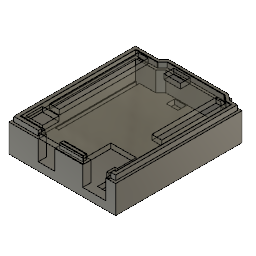
Boîte Arduino V2 F3D (Autodesk Fusion 360 design; units mm, degrees)
Autodesk Fusion 360 part; units mm, degrees
sketch "Esquisse1" plane through (0, 0, 0) normal (0, 0, 1) x (1, 0, 0) in component "Boîte"
  line L0 (-80.3671, -46.9664) -> (-25.3671, -46.9664)
  line L1 (-25.3671, -46.9664) -> (-25.3671, 20.0336)
  line L2 (-80.3671, -46.9664) -> (-80.3671, 20.0336)
  line L3 (-25.3671, 20.0336) -> (-27.7671, 20.0336)
  line L4 (-31.5449, 23.0558) -> (-64.9449, 23.0558)
  line L5 (-67.9671, 20.0336) -> (-80.3671, 20.0336)
  line L6 (-64.9449, 23.0558) -> (-67.9671, 20.0336)
  line L7 (-31.5449, 23.0558) -> (-27.7671, 20.0336)
  line L8 (-85.3671, 25.0336) -> (-85.3671, -51.9664)
  line L9 (-85.3671, -51.9664) -> (-20.3671, -51.9664)
  line L10 (-20.3671, -51.9664) -> (-20.3671, 25.0336)
  line L11 (-20.3671, 25.0336) -> (-26.0132, 25.0336)
  line L12 (-26.0132, 25.0336) -> (-29.791, 28.0558)
  line L13 (-29.791, 28.0558) -> (-67.016, 28.0558)
  line L14 (-67.016, 28.0558) -> (-70.0382, 25.0336)
  line L15 (-70.0382, 25.0336) -> (-85.3671, 25.0336)
  dimension "larg" = 55
  dimension "long" = 67
  dimension "d10" = 67
  dimension "petitcoin" = 2.4
  dimension "d15" = 33.4
  dimension "d18" = 12.4
  dimension "ep" = 5
  dimension "d21" = 5
  dimension "d22" = 5
  dimension "d24" = 5
  dimension "d25" = 5
  dimension "d26" = 5
  dimension "d27" = 5
  dimension "d28" = 5
  constraint horizontal L0
  constraint perpendicular L0 L1
  constraint perpendicular L0 L2
  constraint perpendicular L1 L3
  constraint perpendicular L2 L5
  constraint vertical L8
  constraint perpendicular L8 L9
  constraint perpendicular L9 L10
  constraint perpendicular L10 L11
  constraint perpendicular L10 L13
  constraint perpendicular L8 L15
  constraint parallel L6 L14
  constraint parallel L4 L13
  constraint parallel L7 L12
  measures "larg" distance of L0.start L0.end
  measures "long" distance of L0.end L1.end
  measures "d10" distance of L0.start L2.end
  measures "petitcoin" distance of L1.end L3.end
  measures "d15" distance of L4.start L4.end
  measures "d18" distance of L5.start L2.end
  measures "ep" distance of L2 L8
  measures "d21" distance of L1 L10
  measures "d22" distance of L0 L9
  measures "d24" distance of L6 L14
  measures "d25" distance of L7 L12
  measures "d26" distance of L3 L11
  measures "d27" distance of L4 L13
  measures "d28" distance of L5 L15
sketch "Esquisse2" plane through (0, 0, 0) normal (0, 0, 1) x (1, 0, 0) in component "Boîte"
  line L0 (-26.3671, -46.9664) -> (-40.3671, -46.9664)
  line L1 (-57.3671, -46.9664) -> (-67.3671, -46.9664)
  line L2 (-67.3671, -46.9664) -> (-67.3671, -51.9664)
  line L3 (-57.3671, -46.9664) -> (-57.3671, -51.9664)
  line L4 (-67.3671, -51.9664) -> (-57.3671, -51.9664)
  line L5 (-40.3671, -46.9664) -> (-40.3671, -51.9664)
  line L6 (-26.3671, -46.9664) -> (-26.3671, -51.9664)
  line L7 (-40.3671, -51.9664) -> (-26.3671, -51.9664)
  line L8 (-25.3671, -46.9664) -> (-25.3671, -35.9664)
  line L9 (-25.3671, -35.9664) -> (-36.3671, -35.9664)
  line L10 (-36.3671, -35.9664) -> (-36.3671, -46.9664)
  line L11 (-36.3671, -46.9664) -> (-25.3671, -46.9664)
  line L12 (-25.3671, 20.0336) -> (-25.8671, 20.0336)
  line L13 (-25.8671, 20.0336) -> (-27.8671, 20.0336)
  line L14 (-25.8671, 20.0336) -> (-25.8671, -19.9664)
  line L15 (-27.8671, 20.0336) -> (-27.8671, -19.9664)
  line L16 (-27.8671, -19.9664) -> (-25.8671, -19.9664)
  line L17 (-80.3671, 20.0336) -> (-79.8671, 20.0336)
  line L18 (-79.8671, 20.0336) -> (-77.8671, 20.0336)
  line L19 (-79.8671, 20.0336) -> (-79.8671, -28.9664)
  line L20 (-77.8671, 20.0336) -> (-77.8671, -28.9664)
  line L21 (-79.8671, -28.9664) -> (-77.8671, -28.9664)
  line L22 (-59, 22.5) -> (-52, 22.5)
  line L23 (-59, 22.5) -> (-59, 17.5)
  line L24 (-59, 17.5) -> (-52, 17.5)
  line L25 (-52, 17.5) -> (-52, 22.5)
  point P0 (-25.3671, -46.9664)
  point P1 (-25.3671, 20.0336)
  point P2 (-80.3671, 20.0336)
  dimension "d29" = 1
  dimension "d30" = 14
  dimension "d31" = 17
  dimension "d32" = 10
  dimension "d33" = 5
  dimension "d34" = 5
  dimension "d35" = 5
  dimension "d36" = 5
  dimension "d37" = 11
  dimension "d38" = 11
  dimension "d39" = 11
  dimension "d40" = 0.5
  dimension "d41" = 2
  dimension "d42" = 40
  dimension "d43" = 40
  dimension "d44" = 0.5
  dimension "d45" = 2
  dimension "d46" = 49
  dimension "d47" = 49
  dimension "d50" = 7
  dimension "d51" = 5
  constraint horizontal L0
  constraint perpendicular L1 L2
  constraint perpendicular L1 L3
  constraint perpendicular L0 L5
  constraint perpendicular L0 L6
  constraint coincident P0 L8.start
  constraint perpendicular L7 L8
  constraint perpendicular L8 L9
  constraint perpendicular L9 L10
  constraint coincident P1 L12.start
  constraint horizontal L12
  constraint parallel L12 L13
  constraint perpendicular L12 L14
  constraint perpendicular L13 L15
  constraint coincident P2 L17.start
  constraint horizontal L17
  constraint horizontal L18
  constraint perpendicular L17 L19
  constraint perpendicular L18 L20
  constraint perpendicular L22 L23
  constraint perpendicular L23 L24
  measures "d29" distance of P0 L0.start
  measures "d30" distance of L0.start L0.end
  measures "d31" distance of L0.end L1.start
  measures "d32" distance of L1.start L1.end
  measures "d33" distance of L1.end L2.end
  measures "d34" distance of L1.start L3.end
  measures "d35" distance of L0.end L5.end
  measures "d36" distance of L0.start L6.end
  measures "d37" distance of P0 L8.end
  measures "d38" distance of L8.end L9.end
  measures "d39" distance of L9.end L10.end
  measures "d40" distance of P1 L12.end
  measures "d41" distance of L12.end L13.end
  measures "d42" distance of L12.end L14.end
  measures "d43" distance of L13.end L15.end
  measures "d44" distance of P2 L17.end
  measures "d45" distance of L17.end L18.end
  measures "d46" distance of L17.end L19.end
  measures "d47" distance of L18.end L20.end
  measures "d50" distance of L22.start L22.end
  measures "d51" distance of L22.start L23.end
extrude "Extrusion3" add sketch "Esquisse1" against normal blind 5 contours L0 L1 L2 L3 L4 L5 L6 L7 makes body 1 in component "Boîte"
extrude "Extrusion5" cut sketch "Esquisse2" against normal blind 3 contours L0 L8 L9 L10 L11 | L13 L14 L15 L16 | L18 L19 L20 L21 | L22 L23 L24 L25 bodies 1 in component "Boîte"
extrude "Extrusion6" add sketch "Esquisse1" against normal blind 5 bodies 1 in component "Boîte"
extrude "Extrusion7" add sketch "Esquisse1" along normal blind 12 bodies 1 in component "Boîte"
extrude "Extrusion8" cut sketch "Esquisse2" along normal blind 15 contours L0 L5 L6 L7 L11 | L1 L2 L3 L4 bodies 1 in component "Boîte"
sketch "Esquisse1 (2)" plane through (0, 0, 12) normal (0, 0, 1) x (-1, 0, 0)
  line L0 (67.3671, 51.9664) -> (67.3671, 46.9664)
  line L1 (67.3671, 46.9664) -> (80.3671, 46.9664)
  line L2 (80.3671, 46.9664) -> (80.3671, -20.0336)
  line L3 (80.3671, -20.0336) -> (67.9671, -20.0336)
  line L4 (67.9671, -20.0336) -> (64.9449, -23.0558)
  line L5 (64.9449, -23.0558) -> (31.5449, -23.0558)
  line L6 (31.5449, -23.0558) -> (27.7671, -20.0336)
  line L7 (27.7671, -20.0336) -> (25.3671, -20.0336)
  line L8 (25.3671, -20.0336) -> (25.3671, 46.9664)
  line L9 (25.3671, 46.9664) -> (26.3671, 46.9664)
  line L10 (26.3671, 46.9664) -> (26.3671, 51.9664)
  line L11 (26.3671, 51.9664) -> (20.3671, 51.9664)
  line L12 (20.3671, 51.9664) -> (20.3671, -25.0336)
  line L13 (20.3671, -25.0336) -> (26.0132, -25.0336)
  line L14 (26.0132, -25.0336) -> (29.791, -28.0558)
  line L15 (29.791, -28.0558) -> (67.016, -28.0558)
  line L16 (67.016, -28.0558) -> (70.0382, -25.0336)
  line L17 (70.0382, -25.0336) -> (85.3671, -25.0336)
  line L18 (85.3671, -25.0336) -> (85.3671, 51.9664)
  line L19 (85.3671, 51.9664) -> (67.3671, 51.9664)
  line L20 (83.8671, -20) -> (83.8671, 47)
  line L21 (81.8671, 47) -> (81.8671, -20)
  line L22 (83.8671, 47) -> (83.8671, 50.4664)
  line L23 (83.8671, 50.4664) -> (68.8671, 50.4664)
  line L24 (68.8671, 50.4664) -> (68.8671, 48.4664)
  line L25 (68.8671, 48.4664) -> (81.8671, 48.4664)
  line L26 (81.8671, 48.4664) -> (81.8671, 47)
  line L27 (55.8671, 50.4664) -> (41.8671, 50.4664)
  line L28 (41.8671, 50.4664) -> (41.8671, 48.4664)
  line L29 (41.8671, 48.4664) -> (55.8671, 48.4664)
  line L30 (55.8671, 48.4664) -> (55.8671, 50.4664)
  line L31 (24.8671, 48.4664) -> (24.8671, 50.4664)
  line L32 (24.8671, 50.4664) -> (21.8671, 50.4664)
  line L33 (21.8671, 50.4664) -> (21.8671, -23.5336)
  line L34 (21.8671, -23.5336) -> (26.5394, -23.5336)
  line L35 (26.5394, -23.5336) -> (30.3172, -26.5558)
  line L36 (30.3172, -26.5558) -> (66.3946, -26.5558)
  line L37 (66.3946, -26.5558) -> (69.4169, -23.5336)
  line L38 (69.4169, -23.5336) -> (83.8671, -23.5336)
  line L39 (83.8671, -23.5336) -> (83.8671, -20)
  line L40 (81.8671, -20) -> (81.8671, -21.5336)
  line L41 (81.8671, -21.5336) -> (68.5884, -21.5336)
  line L42 (68.5884, -21.5336) -> (65.5662, -24.5558)
  line L43 (65.5662, -24.5558) -> (31.0187, -24.5558)
  line L44 (31.0187, -24.5558) -> (27.2409, -21.5336)
  line L45 (27.2409, -21.5336) -> (23.8671, -21.5336)
  line L46 (23.8671, -21.5336) -> (23.8671, 48.4664)
  line L47 (23.8671, 48.4664) -> (24.8671, 48.4664)
  line L48 (67.3671, 46.9664) -> (67.3671, 51.9664)
  line L49 (67.3671, 51.9664) -> (57.3671, 51.9664)
  line L50 (57.3671, 46.9664) -> (67.3671, 46.9664)
  line L51 (57.3671, 46.9664) -> (57.3671, 51.9664)
  line L52 (40.3671, 46.9664) -> (40.3671, 51.9664)
  line L53 (26.3671, 46.9664) -> (26.3671, 51.9664)
  line L54 (25.3671, 46.9664) -> (25.3671, 35.9664)
  line L55 (36.3671, 46.9664) -> (25.3671, 46.9664)
  line L56 (25.3671, -20.0336) -> (25.8671, -20.0336)
  dimension "d68" = 1.5
  dimension "distancebord" = 1.5
  dimension "d70" = 1.5
  dimension "d71" = 1.5
  dimension "d72" = 1.5
  dimension "d73" = 1.5
  dimension "d74" = 1.5
  dimension "d75" = 1.5
  dimension "d76" = 1.5
  dimension "d77" = 1.5
  dimension "d78" = 1.5
  dimension "d79" = 1.5
  dimension "d80" = 1.5
  dimension "d81" = 1.5
  dimension "d82" = 1.5
  dimension "d83" = 1.5
  dimension "d84" = 1.5
  dimension "d85" = 1.5
  dimension "d86" = 1.5
  dimension "d87" = 1.5
  dimension "d88" = 1.5
  dimension "d89" = 1.5
  dimension "d90" = 1.5
  dimension "d91" = 1.5
  constraint perpendicular L19 L20
  constraint perpendicular L3 L21
  constraint perpendicular L22 L23
  constraint perpendicular L23 L24
  constraint perpendicular L22 L25
  constraint perpendicular L27 L28
  constraint perpendicular L27 L30
  constraint perpendicular L27 L31
  constraint perpendicular L31 L32
  constraint perpendicular L33 L34
  constraint parallel L17 L36
  constraint parallel L3 L38
  constraint perpendicular L21 L41
  constraint perpendicular L20 L43
  constraint perpendicular L8 L45
  constraint perpendicular L45 L46
  constraint parallel L32 L47
  constraint parallel L12 L33
  constraint parallel L14 L35
  constraint parallel L6 L44
  constraint parallel L16 L37
  constraint parallel L4 L42
  measures "d68" distance of L18 L20
  measures "distancebord" distance of L2 L21
  measures "d70" distance of L1 L25
  measures "d71" distance of L19 L23
  measures "d72" distance of L24 L48
  measures "d73" distance of L27 L49
  measures "d74" distance of L29 L50
  measures "d75" distance of L30 L51
  measures "d76" distance of L28 L52
  measures "d77" distance of L31 L53
  measures "d78" distance of L11 L32
  measures "d79" distance of L12 L33
  measures "d80" distance of L46 L54
  measures "d81" distance of L47 L55
  measures "d82" distance of L13 L34
  measures "d83" distance of L45 L56
  measures "d84" distance of L14 L35
  measures "d85" distance of L6 L44
  measures "d86" distance of L15 L36
  measures "d87" distance of L5 L43
  measures "d88" distance of L16 L37
  measures "d89" distance of L4 L42
  measures "d90" distance of L17 L38
  measures "d91" distance of L3 L41
extrude "Extrusion9" add sketch "Esquisse1 (2)" along normal blind 3 contours L20 L21 L22 L23 L24 L25 L26 L31 L32 L33 L34 L35 L36 L37 L38 L39 L40 L41 L42 L43 L44 L45 L46 L47 | L27 L28 L29 L30 bodies 1 in component "Boîte"
sketch "Esquisse1 (3)" plane through (0, 0, 0) normal (0, 0, 1) x (1, 0, 0) in component "Couvercle"
  line L0 (35.6322, 76.6557) -> (35.6322, 78.6557)
  line L1 (35.6322, 76.6556) -> (35.6322, 78.6559)
  line L2 (4.6323, 75.1557) -> (6.1323, 75.1557)
  line L3 (48.3868, 6.6882) -> (61.6322, 6.6882)
  line L4 (6.1323, 75.1557) -> (6.1323, 80.1558)
  line L5 (3.6323, 76.6) -> (4.7432, 76.6)
  line L6 (7.0061, 6.6549) -> (10.7839, 3.6333)
  line L7 (35.6322, 76.6556) -> (21.6323, 76.6556)
  line L8 (4.7432, 76.6) -> (4.7432, 80.1428)
  line L9 (61.6322, 6.6882) -> (61.6322, 76.5747)
  line L10 (21.6323, 78.6557) -> (21.6323, 76.6557)
  line L11 (50.1322, 75.1557) -> (60.1322, 75.1557)
  line L12 (21.6323, 78.6559) -> (21.6323, 76.6556)
  line L13 (12.1323, 7.6894) -> (6.1323, 7.6894)
  line L14 (12.1323, 46.6558) -> (12.1323, 7.6894)
  line L15 (47.1323, 80.1558) -> (47.1323, 76.5747)
  line L16 (35.6322, 78.6559) -> (21.6323, 78.6559)
  line L17 (3.6323, 6.6549) -> (7.0061, 6.6549)
  line L18 (50.1322, 65.1557) -> (50.1322, 75.1557)
  line L19 (40.3313, 5.1336) -> (30.3313, 5.1336)
  line L20 (30.3313, 5.1336) -> (30.3313, 11.1336)
  line L21 (6.1323, 7.6894) -> (6.1323, 46.6558)
  line L22 (45.3312, 3.6333) -> (48.3868, 6.6882)
  line L23 (53.3822, 7.6894) -> (59.3822, 7.6894)
  line L24 (35.6322, 78.6557) -> (21.6323, 78.6557)
  line L25 (21.6323, 76.6556) -> (35.6322, 76.6556)
  line L26 (60.1322, 65.1557) -> (50.1322, 65.1557)
  line L27 (30.3313, 11.1336) -> (40.3313, 11.1336)
  line L28 (47.1323, 80.1558) -> (4.7432, 80.1558)
  line L29 (21.6323, 76.6557) -> (35.6322, 76.6557)
  line L30 (53.3822, 61.6557) -> (53.3822, 7.6894)
  line L31 (10.7838, 3.6333) -> (45.3312, 3.6333)
  line L32 (20.1324, 78.6559) -> (20.1324, 80.1558)
  line L33 (3.6323, 76.6) -> (3.6323, 6.6549)
  line L34 (40.3313, 11.1336) -> (40.3313, 5.1336)
  line L35 (47.1323, 76.5747) -> (61.6322, 76.5747)
  line L36 (4.6323, 63.6558) -> (4.6323, 75.1557)
  line L37 (35.6322, 76.6556) -> (35.6322, 78.6559)
  line L38 (60.1322, 75.1557) -> (60.1322, 65.1557)
  line L39 (59.3822, 61.6557) -> (53.3822, 61.6557)
  line L40 (20.1324, 78.6559) -> (20.1324, 63.6558)
  line L41 (6.1323, 46.6558) -> (12.1323, 46.6558)
  line L42 (59.3822, 7.6894) -> (59.3822, 61.6557)
  line L43 (20.1324, 63.6558) -> (4.6323, 63.6558)
  constraint coincident L2.start L36
  constraint perpendicular L2 L36
  constraint perpendicular L5 L8
  constraint perpendicular L15 L28
  constraint coincident L15 L35.start
  constraint perpendicular L15 L35
  constraint coincident L9 L35.end
  constraint perpendicular L9 L35
  constraint perpendicular L17 L33
  constraint perpendicular L3 L9
sketch "Esquisse2 (2)" plane through (0, 0, 0) normal (0, 0, 1) x (1, 0, 0) in component "Couvercle"
  line L0 (4.7432, 76.6) -> (4.7432, 80.1428)
  line L1 (4.7432, 80.1428) -> (20.1324, 80.1558)
  line L2 (20.1324, 80.1558) -> (20.1324, 63.6558)
  line L3 (20.1324, 63.6558) -> (4.6323, 63.6558)
  line L4 (20.1324, 80.1558) -> (21.6323, 80.1571)
  line L5 (21.6323, 80.1571) -> (47.1323, 80.1558)
  line L6 (47.1323, 80.1558) -> (47.1323, 76.5747)
  line L7 (47.1323, 76.5747) -> (61.6322, 76.5747)
  line L8 (61.6322, 76.5747) -> (61.6322, 6.6882)
  line L9 (61.6322, 6.6882) -> (48.3868, 6.6882)
  line L10 (48.3868, 6.6882) -> (45.3312, 3.6333)
  line L11 (45.3312, 3.6333) -> (10.7839, 3.6333)
  line L12 (10.7839, 3.6333) -> (7.0061, 6.6549)
  line L13 (7.0061, 6.6549) -> (3.6323, 6.6549)
  line L14 (3.6323, 6.6549) -> (3.6323, 76.6)
  line L15 (3.6323, 76.6) -> (4.7432, 76.6)
  line L16 (30.3313, 11.1336) -> (30.3313, 5.1336)
  line L17 (30.3313, 5.1336) -> (40.3313, 5.1336)
  line L18 (40.3313, 5.1336) -> (40.3313, 11.1336)
  line L19 (40.3313, 11.1336) -> (30.3313, 11.1336)
  line L20 (12.1323, 7.6894) -> (6.1323, 7.6894)
  line L21 (6.1323, 7.6894) -> (6.1323, 46.6558)
  line L22 (6.1323, 46.6558) -> (12.1323, 46.6558)
  line L23 (12.1323, 46.6558) -> (12.1323, 7.6894)
  line L24 (53.3822, 61.6557) -> (59.3822, 61.6557)
  line L25 (59.3822, 61.6557) -> (59.3822, 7.6894)
  line L26 (59.3822, 7.6894) -> (53.3822, 7.6894)
  line L27 (53.3822, 7.6894) -> (53.3822, 61.6557)
  line L28 (50.1322, 75.1557) -> (50.1322, 65.1557)
  line L29 (50.1322, 65.1557) -> (60.1322, 65.1557)
  line L30 (60.1322, 65.1557) -> (60.1322, 75.1557)
  line L31 (60.1322, 75.1557) -> (50.1322, 75.1557)
  line L32 (21.6323, 78.6557) -> (21.6323, 76.6556)
  line L33 (21.6323, 76.6556) -> (35.6322, 76.6557)
  line L34 (35.6322, 76.6557) -> (35.6322, 78.6557)
  line L35 (35.6322, 78.6557) -> (21.6323, 78.6557)
  line L36 (20.1324, 80.1558) -> (47.1323, 80.1558)
  line L37 (6.1323, 75.1557) -> (6.1281, 80.144)
  line L38 (6.1323, 75.1557) -> (4.6323, 75.1557)
  line L39 (4.6323, 75.1557) -> (4.6323, 63.6558)
  point P0 (4.7432, 76.6)
  point P1 (4.7432, 80.1428)
  point P2 (4.6323, 63.6558)
  point P3 (20.1324, 63.6558)
  point P4 (20.1324, 80.1558)
  point P5 (21.6323, 78.6557)
  point P6 (21.6323, 76.6556)
  point P7 (35.6322, 76.6557)
  point P8 (35.6322, 78.6557)
  point P9 (47.1323, 80.1558)
  point P10 (47.1323, 76.5747)
  point P11 (61.6322, 76.5747)
  point P12 (60.1322, 75.1557)
  point P13 (50.1322, 75.1557)
  point P14 (50.1322, 65.1557)
  point P15 (60.1322, 65.1557)
  point P16 (53.3822, 61.6557)
  point P17 (59.3822, 61.6557)
  point P18 (53.3822, 7.6894)
  point P19 (59.3822, 7.6894)
  point P20 (61.6322, 6.6882)
  point P21 (48.3868, 6.6882)
  point P22 (45.3312, 3.6333)
  point P23 (10.7839, 3.6333)
  point P24 (7.0061, 6.6549)
  point P25 (3.6323, 6.6549)
  point P26 (6.1323, 7.6894)
  point P27 (12.1323, 7.6894)
  point P28 (6.1323, 46.6558)
  point P29 (12.1323, 46.6558)
  point P30 (30.3313, 11.1336)
  point P31 (30.3313, 5.1336)
  point P32 (40.3313, 5.1336)
  point P33 (40.3313, 11.1336)
  point P34 (4.6323, 75.1557)
  point P35 (6.1323, 75.1557)
  constraint coincident P0 L0.start
  constraint coincident P1 L0.end
  constraint coincident P4 L1.end
  constraint coincident P3 L2.end
  constraint coincident P2 L3.end
  constraint coincident P9 L5.end
  constraint coincident P10 L6.end
  constraint coincident P11 L7.end
  constraint coincident P20 L8.end
  constraint coincident P21 L9.end
  constraint coincident P22 L10.end
  constraint coincident P23 L11.end
  constraint coincident P24 L12.end
  constraint coincident P25 L13.end
  constraint perpendicular L3 L14
  constraint perpendicular L0 L15
  constraint coincident P30 L16.start
  constraint coincident P31 L16.end
  constraint coincident P32 L17.end
  constraint coincident P33 L18.end
  constraint coincident P27 L20.start
  constraint coincident P26 L20.end
  constraint coincident P28 L21.end
  constraint coincident P29 L22.end
  constraint coincident P16 L24.start
  constraint coincident P17 L24.end
  constraint coincident P19 L25.end
  constraint coincident P18 L26.end
  constraint coincident P13 L28.start
  constraint coincident P14 L28.end
  constraint coincident P15 L29.end
  constraint coincident P12 L30.end
  constraint coincident P5 L32.start
  constraint coincident P6 L32.end
  constraint coincident P7 L33.end
  constraint coincident P8 L34.end
  constraint coincident P35 L37.start
  constraint coincident L1 L37.end
  constraint perpendicular L1 L37
  constraint coincident P34 L38.end
extrude "Extrusion1" add sketch "Esquisse2 (2)" along normal blind 3 separate body contours L0 L1 L2 L3 L4 L5 L6 L7 L8 L9 L10 L11 L12 L13 L14 L15 L36 L37 L38 L39 makes body 2 in component "Couvercle"
move_body "Déplacer1" bodies 2 to x (-1, 0, 0) y (0, -1, 0) z (0, 0, 1) at (0, 0, 0) in component "Couvercle"
move_body "Déplacer2" bodies 2 to x (1, 0, 0) y (0, 1, 0) z (0, 0, 1) at (0, 0, 12) in component "Couvercle"
component "Boîte" placed x (1, 0, 0) y (0, 1, 0) z (0, 0, 1) at (0, 0, 0)
component "Couvercle" placed x (1, 0, 0) y (0, 1, 0) z (0, 0, 1) at (0, 0, 0)
equation "coin = 3.4 mm"
equation "haut = 33.4 mm"
equation "coin2 = 12.4 mm"
equation "d10 = long"
equation "d15 = haut"
equation "d18 = coin2"
equation "d21 = ep"
equation "d22 = ep"
equation "d24 = ep"
equation "d25 = ep"
equation "d26 = ep"
equation "d27 = ep"
equation "d28 = ep"
equation "d33 = ep"
equation "d34 = ep"
equation "d35 = ep"
equation "d36 = ep"
equation "d68 = distancebord"
equation "d70 = distancebord"
equation "d71 = distancebord"
equation "d72 = distancebord"
equation "d73 = distancebord"
equation "d74 = distancebord"
equation "d75 = distancebord"
equation "d76 = distancebord"
equation "d77 = distancebord"
equation "d78 = distancebord"
equation "d79 = distancebord"
equation "d80 = distancebord"
equation "d81 = distancebord"
equation "d82 = distancebord"
equation "d83 = distancebord"
equation "d84 = distancebord"
equation "d85 = distancebord"
equation "d86 = distancebord"
equation "d87 = distancebord"
equation "d88 = distancebord"
equation "d89 = distancebord"
equation "d90 = distancebord"
equation "d91 = distancebord"
